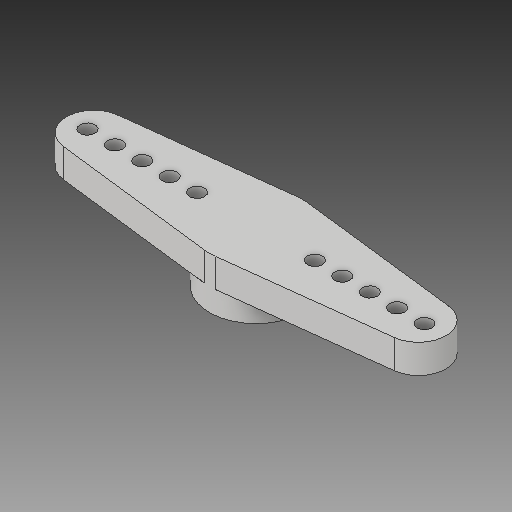
# Autodesk Inventor part: stick
Saved by Autodesk Inventor 2018 (Build 220112000, 112)
## iProperties
Created: 2017-12-10
Part Number: stick
Material: Generic
Document SubType Name: Modeling
Designer: ragna
Density: 1 g/cm^3
Appearance: Default
Author: ragna
Autodesk Inventor part; units mm, degrees
ref_plane "YZ Plane" through (0, 0, 0) normal (1, 0, 0) x (0, 1, 0)
ref_plane "XZ Plane" through (0, 0, 0) normal (0, 1, 0) x (-1, 0, 0)
ref_plane "XY Plane" through (0, 0, 0) normal (0, 0, 1) x (1, 0, 0)
sketch "Sketch1" plane through (0, 0, 0) normal (0, 1, 0) x (-1, 0, 0)
  circle A0 centre (0, 0) radius 3.4
  dimension "d3" = 6.8
  constraints: 1 centre point, 1 coincident
  measures "d3" diameter of A0
extrude "Extrusion1" add sketch "Sketch1" along normal blind 3.75
sketch "Sketch2" plane through (0, 0, 0) normal (0, -1, 0) x (1, 0, 0)
  circle A0 centre (0, 0) radius 2.3583
  constraints: 1 centre point, 1 coincident
extrude "Extrusion2" cut sketch "Sketch2" against normal blind 1.95
sketch "Sketch3" plane through (0, 3.75, 0) normal (0, 1, 0) x (1, 0, 0)
  circle A0 centre (0, 0) radius 3.4 construction
  line L0 (0, -3.4) -> (0, 3.4) construction
  circle A1 centre (-11.85, 0.0077) radius 2
  line L1 (-12.0876, -1.9781) -> (-0.4039, -3.3759)
  line L2 (-12.085, 1.9939) -> (-0.3995, 3.3764)
  circle A2 centre (0, 0) radius 3.4 projected
  dimension "d6" = 4
  dimension "d7" = 11.85
  constraints: 6 end point, 6 point on circle, 4 tangent, 1 centre point, 1 vertical
  measures "d6" diameter of A1
  measures "d7" distance of point (0, 0) A1.centre
extrude "Extrusion3" add sketch "Sketch3" against normal blind 2.1 contours A1 | A1 L2 A2 L1
mirror "Mirror1" about plane through (0, 0, 0) normal (1, 0, 0) of "Extrusion3"
sketch "Sketch4" plane through (0, 3.75, 0) normal (0, 1, 0) x (1, 0, 0)
  circle A0 centre (12.2999, 0) radius 0.55
  arc A1 (12.0876, -1.9781) -> (12.085, 1.9939) centre (11.85, 0.0077) ccw projected
  line L0 (0, 0) -> (13.85, 0) construction
  circle A2 centre (10.2999, 0) radius 0.55
  circle A3 centre (8.2999, 0) radius 0.55
  circle A4 centre (6.2999, 0) radius 0.55
  circle A5 centre (4.2999, 0) radius 0.55
  dimension "d10" = 1.1
  dimension "d11" = 1
  dimension "d14" = 2
  constraints: 5 centre point, 2 end point, 2 horizontal, 1 point on circle, 1 point on line, 8 other
  measures "d10" diameter of A0
  measures "d14" distance of A0.centre A2.centre
extrude "Extrusion4" cut sketch "Sketch4" against normal blind 2.1
mirror "Mirror2" about plane through (0, 0, 0) normal (1, 0, 0) of "Extrusion4"
body "Solid1"
